Autodesk Inventor part; units mm, degrees
(part 2 of 2)
  circle A483 centre (-28.5938, 38.8875) radius 1.994
  circle A484 centre (-33.6737, 38.8875) radius 0.851
  circle A485 centre (-23.5138, 38.8875) radius 0.851
  circle A486 centre (-19.0688, 19.8375) radius 1.994
  circle A487 centre (-24.1488, 19.8375) radius 0.851
  circle A488 centre (-13.9888, 19.8375) radius 0.851
  circle A489 centre (-14.3063, 0.7875) radius 1.994
  circle A490 centre (-19.3863, 0.7875) radius 0.851
  circle A491 centre (-9.2263, 0.7875) radius 0.851
  circle A492 centre (-4.7812, -18.2625) radius 1.994
  circle A493 centre (-9.8613, -18.2625) radius 0.851
  circle A494 centre (0.2988, -18.2625) radius 0.851
  circle A495 centre (-21.45, -37.3125) radius 1.994
  circle A496 centre (-26.53, -37.3125) radius 0.851
  circle A497 centre (-16.37, -37.3125) radius 0.851
  circle A498 centre (-71.488, -30.3275) radius 1.524
  circle A499 centre (28.588, -30.3275) radius 1.524
  circle A500 centre (-71.488, -45.5675) radius 1.994
  circle A501 centre (28.588, -45.5675) radius 1.994
  circle A502 centre (-9.5437, 38.8875) radius 1.994
  circle A503 centre (-14.6237, 38.8875) radius 0.851
  circle A504 centre (-4.4638, 38.8875) radius 0.851
  circle A505 centre (-0.0187, 19.8375) radius 1.994
  circle A506 centre (-5.0987, 19.8375) radius 0.851
  circle A507 centre (5.0613, 19.8375) radius 0.851
  circle A508 centre (4.7438, 0.7875) radius 1.994
  circle A509 centre (-0.3363, 0.7875) radius 0.851
  circle A510 centre (9.8238, 0.7875) radius 0.851
  circle A511 centre (14.2688, -18.2625) radius 1.994
  circle A512 centre (9.1888, -18.2625) radius 0.851
  circle A513 centre (19.3487, -18.2625) radius 0.851
  circle A514 centre (-130.9875, -18.2625) radius 1.994
  circle A515 centre (-136.0675, -18.2625) radius 0.851
  circle A516 centre (-125.9075, -18.2625) radius 0.851
  circle A517 centre (-142.9255, -11.2775) radius 1.524
  circle A518 centre (-119.0495, -11.2775) radius 1.524
  circle A519 centre (-142.9255, -26.5175) radius 1.994
  circle A520 centre (-119.0495, -26.5175) radius 1.994
  circle A521 centre (9.5063, 38.8875) radius 1.994
  circle A522 centre (4.4262, 38.8875) radius 0.851
  circle A523 centre (14.5862, 38.8875) radius 0.851
  circle A524 centre (19.0312, 19.8375) radius 1.994
  circle A525 centre (13.9513, 19.8375) radius 0.851
  circle A526 centre (24.1113, 19.8375) radius 0.851
  circle A527 centre (23.7937, 0.7875) radius 1.994
  circle A528 centre (18.7138, 0.7875) radius 0.851
  circle A529 centre (28.8738, 0.7875) radius 0.851
  circle A530 centre (33.3188, -18.2625) radius 1.994
  circle A531 centre (28.2388, -18.2625) radius 0.851
  circle A532 centre (38.3987, -18.2625) radius 0.851
  circle A533 centre (28.5562, 38.8875) radius 1.994
  circle A534 centre (23.4763, 38.8875) radius 0.851
  circle A535 centre (33.6362, 38.8875) radius 0.851
  circle A536 centre (38.0812, 19.8375) radius 1.994
  circle A537 centre (33.0012, 19.8375) radius 0.851
  circle A538 centre (43.1613, 19.8375) radius 0.851
  circle A539 centre (42.8438, 0.7875) radius 1.994
  circle A540 centre (37.7638, 0.7875) radius 0.851
  circle A541 centre (47.9237, 0.7875) radius 0.851
  circle A542 centre (52.3688, -18.2625) radius 1.994
  circle A543 centre (47.2888, -18.2625) radius 0.851
  circle A544 centre (57.4488, -18.2625) radius 0.851
  circle A545 centre (-140.5125, -37.3125) radius 1.994
  circle A546 centre (-145.5925, -37.3125) radius 0.851
  circle A547 centre (-135.4325, -37.3125) radius 0.851
  circle A548 centre (47.6063, 38.8875) radius 1.994
  circle A549 centre (42.5263, 38.8875) radius 0.851
  circle A550 centre (52.6863, 38.8875) radius 0.851
  circle A551 centre (57.1313, 19.8375) radius 1.994
  circle A552 centre (52.0513, 19.8375) radius 0.851
  circle A553 centre (62.2113, 19.8375) radius 0.851
  circle A554 centre (61.8937, 0.7875) radius 1.994
  circle A555 centre (56.8137, 0.7875) radius 0.851
  circle A556 centre (66.9737, 0.7875) radius 0.851
  circle A557 centre (71.4188, -18.2625) radius 1.994
  circle A558 centre (66.3388, -18.2625) radius 0.851
  circle A559 centre (76.4988, -18.2625) radius 0.851
  circle A560 centre (47.6063, -37.3125) radius 1.994
  circle A561 centre (42.5263, -37.3125) radius 0.851
  circle A562 centre (52.6863, -37.3125) radius 0.851
  circle A563 centre (66.6562, 38.8875) radius 1.994
  circle A564 centre (61.5763, 38.8875) radius 0.851
  circle A565 centre (71.7362, 38.8875) radius 0.851
  circle A566 centre (76.1813, 19.8375) radius 1.994
  circle A567 centre (71.1012, 19.8375) radius 0.851
  circle A568 centre (81.2613, 19.8375) radius 0.851
  circle A569 centre (80.9437, 0.7875) radius 1.994
  circle A570 centre (75.8638, 0.7875) radius 0.851
  circle A571 centre (86.0238, 0.7875) radius 0.851
  circle A572 centre (97.6125, -18.2625) radius 1.994
  circle A573 centre (92.5325, -18.2625) radius 0.851
  circle A574 centre (102.6925, -18.2625) radius 0.851
  circle A575 centre (-123.8438, 38.8875) radius 1.994
  circle A576 centre (-128.9238, 38.8875) radius 0.851
  circle A577 centre (-118.7638, 38.8875) radius 0.851
  circle A578 centre (66.6562, -37.3125) radius 1.994
  circle A579 centre (61.5763, -37.3125) radius 0.851
  circle A580 centre (71.7362, -37.3125) radius 0.851
  circle A581 centre (85.7062, 38.8875) radius 1.994
  circle A582 centre (80.6262, 38.8875) radius 0.851
  circle A583 centre (90.7863, 38.8875) radius 0.851
  circle A584 centre (95.2313, 19.8375) radius 1.994
  circle A585 centre (90.1513, 19.8375) radius 0.851
  circle A586 centre (100.3113, 19.8375) radius 0.851
  circle A587 centre (111.9, 0.7875) radius 1.994
  circle A588 centre (106.82, 0.7875) radius 0.851
  circle A589 centre (116.98, 0.7875) radius 0.851
  circle A590 centre (99.962, 7.7725) radius 1.524
  circle A591 centre (123.838, 7.7725) radius 1.524
  circle A592 centre (99.962, -7.4675) radius 1.994
  circle A593 centre (123.838, -7.4675) radius 1.994
  circle A594 centre (123.8063, -18.2625) radius 1.994
  circle A595 centre (118.7262, -18.2625) radius 0.851
  circle A596 centre (128.8862, -18.2625) radius 0.851
  circle A597 centre (85.7062, -37.3125) radius 1.994
  circle A598 centre (80.6262, -37.3125) radius 0.851
  circle A599 centre (90.7863, -37.3125) radius 0.851
  circle A600 centre (114.2813, 38.8875) radius 1.994
  circle A601 centre (109.2013, 38.8875) radius 0.851
  circle A602 centre (119.3613, 38.8875) radius 0.851
  circle A603 centre (102.3432, 45.8725) radius 1.524
  circle A604 centre (126.2193, 45.8725) radius 1.524
  circle A605 centre (102.3432, 30.6325) radius 1.994
  circle A606 centre (126.2193, 30.6325) radius 1.994
  circle A607 centre (119.0438, 19.8375) radius 1.994
  circle A608 centre (113.9638, 19.8375) radius 0.851
  circle A609 centre (124.1238, 19.8375) radius 0.851
  circle A610 centre (142.8562, 0.7875) radius 1.994
  circle A611 centre (137.7763, 0.7875) radius 0.851
  circle A612 centre (147.9363, 0.7875) radius 0.851
  circle A613 centre (142.8562, -18.2625) radius 1.994
  circle A614 centre (137.7763, -18.2625) radius 0.851
  circle A615 centre (147.9363, -18.2625) radius 0.851
  circle A616 centre (-114.3187, 19.8375) radius 1.994
  circle A617 centre (-119.3988, 19.8375) radius 0.851
  circle A618 centre (-109.2388, 19.8375) radius 0.851
  circle A619 centre (123.8063, -37.3125) radius 1.994
  circle A620 centre (118.7262, -37.3125) radius 0.851
  circle A621 centre (128.8862, -37.3125) radius 0.851
  circle A622 centre (142.8562, 38.8875) radius 1.994
  circle A623 centre (137.7763, 38.8875) radius 0.851
  circle A624 centre (147.9363, 38.8875) radius 0.851
  circle A625 centre (142.8562, 19.8375) radius 1.994
  circle A626 centre (137.7763, 19.8375) radius 0.851
  circle A627 centre (147.9363, 19.8375) radius 0.851
  circle A628 centre (104.7563, -37.3125) radius 1.994
  circle A629 centre (99.6762, -37.3125) radius 0.851
  circle A630 centre (109.8363, -37.3125) radius 0.851
  circle A631 centre (142.8562, -37.3125) radius 1.994
  circle A632 centre (137.7763, -37.3125) radius 0.851
  circle A633 centre (147.9363, -37.3125) radius 0.851
  circle A634 centre (-109.5563, 0.7875) radius 1.994
  circle A635 centre (-114.6363, 0.7875) radius 0.851
  circle A636 centre (-104.4763, 0.7875) radius 0.851
  circle A637 centre (-100.0312, -18.2625) radius 1.994
  circle A638 centre (-105.1112, -18.2625) radius 0.851
  circle A639 centre (-94.9513, -18.2625) radius 0.851
  constraints: 640 centre point, 562 end point, 560 point on circle
extrude "60pc_pcb.kicad_pcb_Outline" add sketch "Sketch1" along normal blind 1.6
sketch "Sketch2" plane through (0, 0, 1.6) normal (0, 0, 1) x (1, 0, 0)
  point P0 (0, 0)
body "Solid1"
